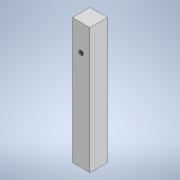
# Autodesk Inventor part: Suport_Cam
Saved by Autodesk Inventor 2021 (Build 250183000, 183)
## iProperties
Created: 2021-06-02
Part Number: Suport_Cam
Material: Genérico
Document SubType Name: Modeling
Designer: Marc
Density: 1 g/cm^3
Appearance: Valor por defecto
Author: Marc
Autodesk Inventor part; units mm, degrees
ref_plane "YZ Plane" through (0, 0, 0) normal (1, 0, 0) x (0, 1, 0)
ref_plane "XZ Plane" through (0, 0, 0) normal (0, 1, 0) x (-1, 0, 0)
ref_plane "XY Plane" through (0, 0, 0) normal (0, 0, 1) x (1, 0, 0)
sketch "Boceto1" plane through (0, 0, 0) normal (0, 0, 1) x (1, 0, 0)
  line L0 (-10, -71.5) -> (10, -71.5)
  line L1 (10, -71.5) -> (10, 71.5)
  line L2 (10, 71.5) -> (-10, 71.5)
  line L3 (-10, 71.5) -> (-10, -71.5)
  line L4 (-10, -71.5) -> (10, 71.5) construction
  line L5 (10, -71.5) -> (-10, 71.5) construction
  point P0 (0, 0)
  dimension "d0" = 20
  dimension "d1" = 143
  constraints: 12 end point, 2 midpoint, 2 parallel, 1 horizontal, 1 perpendicular
  measures "d0" distance of L2.end L1.end
  measures "d1" distance of L1.end L0.end
extrude "Extrusión1" add sketch "Boceto1" against normal blind 20
sketch "Boceto2" plane through (0, 0, 0) normal (0, 0, 1) x (1, 0, 0)
  line L0 (-10, 71.5) -> (10, 71.5) projected
  circle A0 centre (0, 41.5) radius 2.5
  point P0 (0, 0)
  dimension "d5" = 5
  constraints: 1 centre point
  measures "d5" diameter of A0
extrude "Extrusión2" cut sketch "Boceto2" against normal blind 10
thread "Rosca1" size "M5x0.8" class "6H" standard "ANSI Metric M Profile" full length
sketch "Boceto3" plane through (-10, -71.5, 0) normal (0, -1, 0) x (1, 0, 0)
  circle A0 centre (10, -10) radius 2.5
  point P0 (10, 0)
  constraints: 1 centre point
extrude "Extrusión3" cut sketch "Boceto3" against normal blind 10
thread "Rosca2" size "M5x0.8" class "6H" standard "ANSI Metric M Profile" full length
